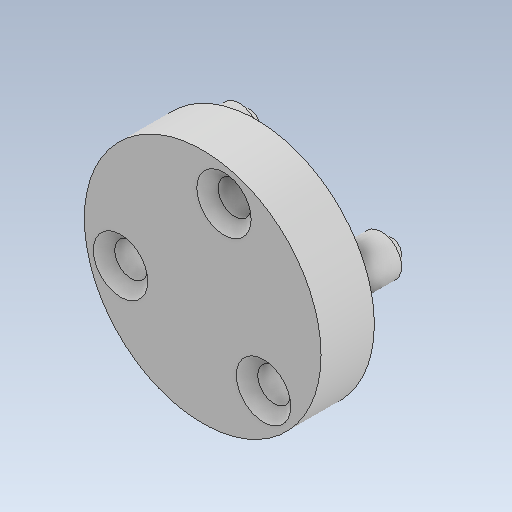
# Autodesk Inventor part: ВедущееКолесоВнутр
Saved by Autodesk Inventor 2020 (Build 240168000, 168)
## iProperties
Created: 2021-03-04
Part Number: ВедущееКолесоВнутр
Material: Типовые
Document SubType Name: Modeling
Designer: I_Love_U_Bogdan
Density: 1 g/cm^3
Appearance: По умолчанию
Author: I_Love_U_Bogdan
Autodesk Inventor part; units mm, degrees
ref_plane "YZ Plane" through (0, 0, 0) normal (1, 0, 0) x (0, 1, 0)
ref_plane "XZ Plane" through (0, 0, 0) normal (0, 1, 0) x (-1, 0, 0)
ref_plane "XY Plane" through (0, 0, 0) normal (0, 0, 1) x (1, 0, 0)
sketch "Эскиз1" plane through (0, 0, 0) normal (0, 0, 1) x (1, 0, 0)
  circle A0 centre (0, 0) radius 11.3
  circle A1 centre (-7.7068, -2.1459) radius 1.55
  circle A2 centre (1.995, 7.7473) radius 1.55
  circle A3 centre (-7.7068, -2.1459) radius 1.55
  circle A4 centre (1.995, 7.7473) radius 1.55
  circle A5 centre (5.7118, -5.6014) radius 1.55
  circle A6 centre (0, 0) radius 11.3
  circle A7 centre (7.7568, 1.9574) radius 2
  circle A8 centre (-2.1832, -7.6963) radius 2
  circle A9 centre (-5.5736, 5.7389) radius 2
  circle A10 centre (0, 0) radius 11.1
  point P0 (0, 0)
extrude "Выдавливание1" add sketch "Эскиз1" along normal blind 5 contours A7 | A8 | A9 | A10
sketch "Эскиз2" plane through (0, 0, 0) normal (0, 0, -1) x (-1, 0, 0)
  circle A0 centre (5.5736, 5.7389) radius 2 projected
  circle A1 centre (2.1832, -7.6963) radius 2 projected
  circle A2 centre (-7.7568, 1.9574) radius 2 projected
  circle A3 centre (5.5736, 5.7389) radius 1.9
  circle A4 centre (2.1832, -7.6963) radius 1.9
  circle A5 centre (-7.7568, 1.9574) radius 1.9
  point P0 (0, 0)
  dimension "d3" = 0.1
  dimension "d4" = 0.1
  dimension "d5" = 0.1
  constraints: 3 centre point
  measures "d3" radial gap between concentric circles of A0 A3
  measures "d4" radial gap between concentric circles of A1 A4
  measures "d5" radial gap between concentric circles of A2 A5
extrude "Выдавливание2" add sketch "Эскиз2" along normal blind 5 contours A3 | A4 | A5
chamfer "Фаска1" distance 1 angle 45 6 edges at (9.6568, 1.9574, -5) (-3.6736, 5.7389, -5) (-0.2832, -7.6963, -5) (4.1618, -5.6014, 5) (0.445, 7.7473, 5) (-9.2568, -2.1459, 5)
